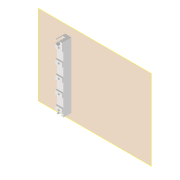
# Autodesk Inventor part: Omniscope_USBC_Bar
Saved by Autodesk Inventor 2022 (Build 260153000, 153)
## iProperties
Created: 2023-05-17
Part Number: Omniscope_USBC_Bar
Material: Generisch
Document SubType Name: Modeling
Designer: diederichbenedict
Density: 1 g/cm^3
Appearance: Vorgabe
Author: diederichbenedict
Autodesk Inventor part; units mm, degrees
ref_plane "YZ Plane" through (0, 0, 0) normal (1, 0, 0) x (0, 1, 0)
ref_plane "XZ Plane" through (0, 0, 0) normal (0, 1, 0) x (-1, 0, 0)
ref_plane "Arbeitsebene1" through (0, 0, 0) normal (0, 0, 1) x (1, 0, 0)
sketch "Skizze1" plane through (0, 0, 0) normal (0, 0, 1) x (1, 0, 0)
  line L0 (-69.421, 36.3204) -> (-72.421, 39.3204) projected
  line L1 (-69.421, 36.3204) -> (-60.421, 36.3204) projected
  line L2 (-57.421, 33.3204) -> (-60.421, 36.3204) projected
  line L3 (-57.421, 33.3204) -> (-57.421, -36.5796) projected
  line L4 (-60.421, -39.5796) -> (-57.421, -36.5796) projected
  line L5 (-60.421, -39.5796) -> (-69.421, -39.5796) projected
  line L6 (-72.421, -42.5796) -> (-69.421, -39.5796) projected
  line L7 (-72.421, -42.5796) -> (-72.421, -47.4152) projected
  arc A0 (-72.421, -47.4152) -> (-68.421, -51.4152) centre (-68.421, -47.4152) ccw projected
  line L8 (-68.421, -51.4152) -> (68.421, -51.4152) projected
  arc A1 (68.421, -51.4152) -> (72.421, -47.4152) centre (68.421, -47.4152) ccw projected
  line L9 (72.421, -47.4152) -> (72.421, -42.5796) projected
  line L10 (69.421, -39.5796) -> (72.421, -42.5796) projected
  line L11 (69.421, -39.5796) -> (65.421, -39.5796) projected
  line L12 (62.421, -36.5796) -> (65.421, -39.5796) projected
  line L13 (62.421, -36.5796) -> (62.421, 33.3204) projected
  line L14 (65.421, 36.3204) -> (62.421, 33.3204) projected
  line L15 (65.421, 36.3204) -> (69.421, 36.3204) projected
  line L16 (72.421, 39.3204) -> (69.421, 36.3204) projected
  line L17 (72.421, 39.3204) -> (72.421, 47.4152) projected
  arc A2 (72.421, 47.4152) -> (68.421, 51.4152) centre (68.421, 47.4152) ccw projected
  line L18 (68.421, 51.4152) -> (-68.421, 51.4152) projected
  arc A3 (-68.421, 51.4152) -> (-72.421, 47.4152) centre (-68.421, 47.4152) ccw projected
  line L19 (-72.421, 47.4152) -> (-72.421, 39.3204) projected
  circle A4 centre (68.921, 47.9152) radius 1.4 projected
  circle A5 centre (68.921, -47.9152) radius 1.4 projected
  circle A6 centre (-68.921, -47.9152) radius 1.4 projected
  circle A7 centre (-68.921, 47.9152) radius 1.5 projected
  circle A8 centre (-38.7933, -44.5796) radius 1.4 projected
  circle A9 centre (-38.7933, 41.3204) radius 1.4 projected
  line L20 (-48.1034, 36.3204) -> (-38.1034, 36.3204) projected
  line L21 (-38.1034, 36.3204) -> (-38.1034, -39.5796) projected
  line L22 (-38.1034, -39.5796) -> (-48.1034, -39.5796) projected
  line L23 (-48.1034, -39.5796) -> (-48.1034, 36.3204) projected
  circle A10 centre (-20.0933, 41.3204) radius 1.4 projected
  circle A11 centre (-20.0933, -44.5796) radius 1.4 projected
  line L24 (-19.4034, -39.5796) -> (-29.4034, -39.5796) projected
  line L25 (-29.4034, -39.5796) -> (-29.4034, 36.3204) projected
  line L26 (-29.4034, 36.3204) -> (-19.4034, 36.3204) projected
  line L27 (-19.4034, 36.3204) -> (-19.4034, -39.5796) projected
  circle A12 centre (-1.3933, 41.3204) radius 1.4 projected
  circle A13 centre (-1.3933, -44.5796) radius 1.4 projected
  line L28 (-0.7034, -39.5796) -> (-10.7034, -39.5796) projected
  line L29 (-10.7034, -39.5796) -> (-10.7034, 36.3204) projected
  line L30 (-10.7034, 36.3204) -> (-0.7034, 36.3204) projected
  line L31 (-0.7034, 36.3204) -> (-0.7034, -39.5796) projected
  circle A14 centre (17.3067, 41.3204) radius 1.4 projected
  circle A15 centre (17.3067, -44.5796) radius 1.4 projected
  line L32 (17.9966, -39.5796) -> (7.9966, -39.5796) projected
  line L33 (7.9966, -39.5796) -> (7.9966, 36.3204) projected
  line L34 (7.9966, 36.3204) -> (17.9966, 36.3204) projected
  line L35 (17.9966, 36.3204) -> (17.9966, -39.5796) projected
  circle A16 centre (36.0067, 41.3204) radius 1.4 projected
  circle A17 centre (36.0067, -44.5796) radius 1.4 projected
  line L36 (36.6966, -39.5796) -> (26.6966, -39.5796) projected
  line L37 (26.6966, -39.5796) -> (26.6966, 36.3204) projected
  line L38 (26.6966, 36.3204) -> (36.6966, 36.3204) projected
  line L39 (36.6966, 36.3204) -> (36.6966, -39.5796) projected
  circle A18 centre (54.7067, 41.3204) radius 1.4 projected
  circle A19 centre (54.7067, -44.5796) radius 1.4 projected
  line L40 (55.3966, -39.5796) -> (45.3966, -39.5796) projected
  line L41 (45.3966, -39.5796) -> (45.3966, 36.3204) projected
  line L42 (45.3966, 36.3204) -> (55.3966, 36.3204) projected
  line L43 (55.3966, 36.3204) -> (55.3966, -39.5796) projected
  line L44 (-32.7933, 44.3204) -> (-41.7933, 44.3204)
  line L45 (-41.7933, 44.3204) -> (-41.7933, -47.5796)
  line L46 (-41.7933, -47.5796) -> (-32.7933, -47.5796)
  line L47 (-32.7933, -47.5796) -> (-32.7933, 44.3204)
  circle A20 centre (-37.2933, 36.3204) radius 1.4
  circle A21 centre (-37.2933, -39.5796) radius 1.4
  point P0 (0, 0)
  dimension "d0" = 3
  dimension "d1" = 3
  dimension "d2" = 3
  dimension "d3" = 6
  dimension "d4" = 2.8
  dimension "d5" = 2.8
  constraints: 8 end point, 2 centre point, 2 parallel, 1 horizontal, 1 perpendicular
  measures "d0" distance from line of A9.centre L44
  measures "d1" distance from line of L46 A8.centre
  measures "d2" distance from line of A8.centre L45
  measures "d3" distance from line of A8.centre L47
  measures "d4" diameter of A20
  measures "d5" diameter of A21
ref_plane "Arbeitsebene2" through (-44.2034, 20.4204, 13.5) normal (0, 0, -1) x (0, 1, 0)
extrude "Extrusion1" add sketch "Skizze1" along normal up to surface (13.5 mm away) contours L45 L44 L47 L46 L22 A21 L21 A20 L20 | L20 A20 L21 A21 L22 L45
sketch "Skizze2" plane through (-41.7933, -47.5796, 13.5) normal (0, 0, 1) x (1, 0, 0)
  line L0 (9, 68) -> (-3, 68) projected
  line L1 (-3, 80) -> (9, 80) projected
  line L2 (-3, 61.3) -> (9, 61.3) projected
  line L3 (9, 49.3) -> (-3, 49.3) projected
  line L4 (-3, 42.6) -> (9, 42.6) projected
  line L5 (9, 30.6) -> (-3, 30.6) projected
  line L6 (-3, 23.9) -> (9, 23.9) projected
  line L7 (9, 11.9) -> (-3, 11.9) projected
  line L8 (9, 80) -> (-3, 80)
  line L9 (-3, 80) -> (-3, 68)
  line L10 (-3, 68) -> (9, 68)
  line L11 (9, 68) -> (9, 80)
  line L12 (-3.2, 67.8) -> (-3.2, 80.2)
  line L13 (-3.2, 80.2) -> (9.2, 80.2)
  line L14 (9.2, 80.2) -> (9.2, 67.8)
  line L15 (9.2, 67.8) -> (-3.2, 67.8)
  point P0 (41.7933, 47.5796)
  dimension "d8" = 0.2
  constraints: 16 end point, 4 parallel, 2 perpendicular, 1 horizontal, 3 other
  measures "d8" distance between parallel lines of L9 L12
extrude "Extrusion2" cut sketch "Skizze2" against normal blind 2 contours L0 L9 L1 L11 | L12 L13 L14 L15
pattern_linear "Rechteckige Anordnung1" count 5 spacing 18.7 along (0, -1, 0) of "Extrusion2"
sketch "Skizze3" plane through (-41.7933, 20.2204, 13.5) normal (0, 0, 1) x (1, 0, 0)
  line L0 (0, -6.3) -> (9, -6.3) projected
  line L1 (9, -6.3) -> (9, 0) projected
  line L2 (9, 0) -> (0, 0) projected
  line L3 (0, 0) -> (0, -6.3) projected
  line L4 (0, -25) -> (9, -25) projected
  line L5 (9, -25) -> (9, -18.7) projected
  line L6 (9, -18.7) -> (0, -18.7) projected
  line L7 (0, -18.7) -> (0, -25) projected
  line L8 (0, -43.7) -> (9, -43.7) projected
  line L9 (9, -43.7) -> (9, -37.4) projected
  line L10 (9, -37.4) -> (0, -37.4) projected
  line L11 (0, -37.4) -> (0, -43.7) projected
  circle A0 centre (4.5, -3.15) radius 1.4
  circle A1 centre (4.5, -21.85) radius 1.4
  circle A2 centre (4.5, -40.55) radius 1.4
  point P0 (41.7933, -20.2204)
  dimension "d14" = 2.8
  dimension "d15" = 2.8
  dimension "d16" = 2.8
  constraints: 3 centre point
  measures "d14" diameter of A0
  measures "d15" diameter of A1
  measures "d16" diameter of A2
extrude "Extrusion3" cut sketch "Skizze3" against normal through all contours A0 | A1 | A2
sketch "Skizze4" plane through (-41.7933, -42.1796, 13.5) normal (0, 0, 1) x (1, 0, 0)
  circle A0 centre (3, 83.5) radius 1.4 projected
  circle A1 centre (4.5, 78.5) radius 1.4 projected
  line L0 (0, 74.8) -> (9, 74.8) projected
  line L1 (9, 74.8) -> (9, 86.5) projected
  line L2 (9, 86.5) -> (0, 86.5) projected
  line L3 (0, 86.5) -> (0, 74.8) projected
  line L4 (9, 0) -> (9, -5.4) projected
  line L5 (0, 0) -> (9, 0) projected
  line L6 (0, -5.4) -> (0, 0) projected
  line L7 (9, -5.4) -> (0, -5.4) projected
  circle A2 centre (3, -2.4) radius 1.4 projected
  point P0 (41.7933, 42.1796)
hole "Bohrung1" at (-38.7933, 41.3204, 13.5) at (-38.7933, -44.5796, 13.5) direction (0, 0, -1) diameter 3.2 end through all counterbore diameter 7 counterbore depth 9
